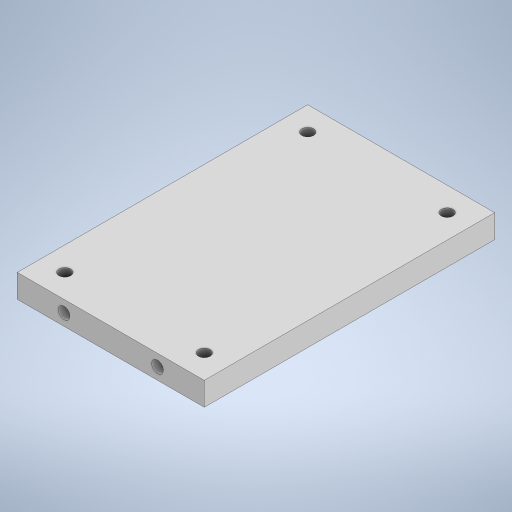
# Autodesk Inventor part: FloorMountV2
Saved by Autodesk Inventor 2024 (Build 280153000, 153)
## iProperties
Created: 2024-03-22
Part Number: FloorMountV2
Material: Generic
Document SubType Name: Modeling
Designer: yusuf
Density: 1 g/cm^3
Appearance: Default
Author: yusuf
Autodesk Inventor part; units mm, degrees
ref_plane "YZ Plane" through (0, 0, 0) normal (1, 0, 0) x (0, 1, 0)
ref_plane "XZ Plane" through (0, 0, 0) normal (0, 1, 0) x (-1, 0, 0)
ref_plane "XY Plane" through (0, 0, 0) normal (0, 0, 1) x (1, 0, 0)
sketch "Sketch1" plane through (0, 0, 0) normal (0, 1, 0) x (-1, 0, 0)
  line L0 (0, 0) -> (199.9996, 0)
  line L1 (199.9996, 0) -> (199.9996, -310.5912)
  line L2 (199.9996, -310.5912) -> (0, -310.5912)
  line L3 (0, -310.5912) -> (0, 0)
  dimension "d0" = 199.9996
  dimension "d1" = 310.5912
  constraints: 8 end point, 2 parallel, 1 horizontal, 1 perpendicular
  measures "d0" distance of L1.end L2.end
  measures "d1" distance of L0.end L1.end
extrude "Extrusion1" add sketch "Sketch1" along normal blind 24.9936
sketch "Sketch2" plane through (0, 24.9936, 0) normal (0, 1, 0) x (1, 0, 0)
  circle A0 centre (-174.5996, 25.4) radius 6.35
  circle A1 centre (-174.5996, 285.1912) radius 6.35
  circle A2 centre (-25.4, 25.4) radius 6.35
  circle A3 centre (-25.4, 285.1912) radius 6.35
  line L0 (-199.9996, 310.5912) -> (-199.9996, 0) projected
  line L1 (-199.9996, 0) -> (0, 0) projected
  line L2 (0, 310.5912) -> (-199.9996, 310.5912) projected
  line L3 (0, 0) -> (0, 310.5912) projected
  dimension "d4" = 12.7
  dimension "d5" = 25.4
  dimension "d6" = 25.4
  dimension "d7" = 12.7
  dimension "d8" = 25.4
  dimension "d9" = 25.4
  dimension "d10" = 25.4
  dimension "d11" = 25.4
  dimension "d12" = 12.7
  dimension "d13" = 12.7
  dimension "d14" = 25.4
  dimension "d15" = 25.4
  constraints: 4 centre point
  measures "d4" diameter of A0
  measures "d5" distance from line of A0.centre L0
  measures "d6" distance from line of L1 A0.centre
  measures "d7" diameter of A1
  measures "d8" distance from line of L0 A1.centre
  measures "d9" distance from line of L2 A1.centre
  measures "d10" distance from line of L2 A3.centre
  measures "d11" distance from line of L3 A3.centre
  measures "d12" diameter of A3
  measures "d13" diameter of A2
  measures "d14" distance from line of L1 A2.centre
  measures "d15" distance from line of L3 A2.centre
extrude "Extrusion2" cut sketch "Sketch2" against normal blind 24.9936 contours A0 | A1 | A2 | A3
sketch "Sketch3" plane through (-199.9996, 0, 0) normal (0, 0, 1) x (1, 0, 0)
  circle A0 centre (50, 12.4968) radius 6.35
  circle A1 centre (149.9996, 12.4968) radius 6.35
  line L0 (0, 0) -> (0, 24.9936) projected
  line L1 (0, 24.9936) -> (199.9996, 24.9936) projected
  line L2 (199.9996, 0) -> (199.9996, 24.9936) projected
  point P0 (199.9996, 12.4968)
  dimension "d18" = 12.7
  dimension "d19" = 50
  dimension "d20" = 12.4968
  dimension "d21" = 12.4968
  dimension "d22" = 50
  dimension "d23" = 12.7
  constraints: 2 centre point, 1 midpoint
  measures "d18" diameter of A0
  measures "d19" distance from line of L0 A0.centre
  measures "d20" distance from line of L1 A0.centre
  measures "d21" distance from line of L1 A1.centre
  measures "d22" distance of point (200, 12.497) A1.centre
  measures "d23" diameter of A1
sketch "Sketch4" plane through (0, 0, -310.5912) normal (0, 0, -1) x (-1, 0, 0)
  circle A0 centre (50, 12.4968) radius 6.35
  circle A1 centre (149.9996, 12.4968) radius 6.35
  line L0 (0, 0) -> (0, 24.9936) projected
  line L1 (0, 0) -> (199.9996, 0) projected
  line L2 (199.9996, 0) -> (199.9996, 24.9936) projected
  dimension "d24" = 12.7
  dimension "d25" = 12.7
  dimension "d26" = 50
  dimension "d27" = 12.4968
  dimension "d28" = 12.4968
  dimension "d29" = 50
  constraints: 2 centre point
  measures "d24" diameter of A1
  measures "d25" diameter of A0
  measures "d26" distance from line of L0 A0.centre
  measures "d27" distance from line of L1 A0.centre
  measures "d28" distance from line of L1 A1.centre
  measures "d29" distance from line of L2 A1.centre
extrude "Extrusion3" cut sketch "Sketch3" against normal blind 20
extrude "Extrusion4" cut sketch "Sketch4" against normal blind 20
equation "\"d7\" = d4"
equation "\"d8\" = d5"
equation "\"d9\" = d5"
equation "\"d10\" = d5"
equation "\"d11\" = d5"
equation "\"d12\" = d4"
equation "\"d13\" = d4"
equation "\"d14\" = d5"
equation "\"d15\" = d5"
equation "\"d21\" = d20"
equation "\"d22\" = d19"
equation "\"d23\" = d18"
equation "\"d24\" = d18"
equation "\"d25\" = d18"
equation "\"d26\" = d22"
equation "\"d27\" = d21"
equation "\"d28\" = d21"
equation "\"d29\" = d26"
body "Solid1"
